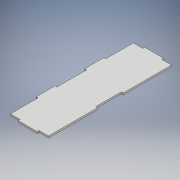
# Autodesk Inventor part: sampingkiri
Saved by Autodesk Inventor 2017 (Build 210142000, 142)
## iProperties
Created: 2017-01-17
Part Number: sampingkiri
Material: Generic
Document SubType Name: Modeling
Designer: Ghesa Bhakti
Density: 1 g/cm^3
Appearance: Default
Author: Ghesa Bhakti
Autodesk Inventor part; units mm, degrees
ref_plane "YZ Plane" through (0, 0, 0) normal (1, 0, 0) x (0, 1, 0)
ref_plane "XZ Plane" through (0, 0, 0) normal (0, 1, 0) x (-1, 0, 0)
ref_plane "XY Plane" through (0, 0, 0) normal (0, 0, 1) x (1, 0, 0)
sketch "Sketch1" plane through (0, 0, 0) normal (0, 0, 1) x (1, 0, 0)
  line L0 (60.0759, 197.5616) -> (45.0759, 197.5616)
  line L1 (45.0759, 197.5616) -> (45.0759, 200.5616)
  line L2 (15.0759, 200.5616) -> (15.0759, 197.5616)
  line L3 (45.0759, 200.5616) -> (15.0759, 200.5616)
  line L4 (15.0759, 197.5616) -> (0.0759, 197.5616)
  line L5 (57.0759, 81.5616) -> (60, 81.5616)
  line L6 (0.0759, 77.6616) -> (-2.9241, 77.6616)
  line L7 (-2.9241, 77.6616) -> (-2.9241, 47.8616)
  line L8 (-2.9241, 47.8616) -> (0.0759, 47.8616)
  line L9 (60, 4.5616) -> (60, 81.5616)
  line L10 (0.0759, 47.8616) -> (0.0759, 4.5616)
  line L11 (0.0759, 4.5616) -> (15.0759, 4.5616)
  line L12 (60.0757, 4.4159) -> (60, 4.5616)
  line L13 (45.0759, 4.4159) -> (60.0757, 4.4159)
  line L14 (45.0759, 4.4159) -> (45.0759, 1.4159)
  line L15 (45.0759, 1.4159) -> (15.0759, 1.5616)
  line L16 (15.0759, 1.5616) -> (15.0759, 4.5616)
  line L17 (0.0759, 197.5616) -> (0.0759, 154.2616)
  line L18 (0.0759, 154.2616) -> (-2.9241, 154.2616)
  line L19 (60.0759, 121.5616) -> (60.0759, 197.5616)
  line L20 (60.0759, 121.5616) -> (57.0759, 121.5616)
  line L21 (-2.9241, 124.2616) -> (0.0759, 124.2616)
  line L22 (-2.9241, 154.2616) -> (-2.9241, 124.2616)
  line L23 (0.0759, 124.2616) -> (0.0759, 77.6616)
  line L24 (57.0759, 121.5616) -> (57.0759, 81.5616)
  point P0 (0, 0)
  dimension "d47" = 193
  dimension "d48" = 60
  dimension "d49" = 3
  dimension "d50" = 30
  dimension "d51" = 15
  dimension "d52" = 3
  dimension "d53" = 3
  dimension "d54" = 15
  dimension "d55" = 3
  dimension "d56" = 3
  dimension "d57" = 3
  dimension "d58" = 3
  dimension "d59" = 15
  dimension "d60" = 40
  dimension "d61" = 3
  dimension "d62" = 77
  dimension "d63" = 3
  dimension "d64" = 76
  dimension "d65" = 199.1457
  dimension "d66" = 43.3
  dimension "d67" = 46.6
  dimension "d68" = 43.3
  dimension "d69" = 30
  dimension "d70" = 29.8
  constraints: 50 end point, 9 parallel, 5 horizontal, 3 perpendicular, 2 vertical, 1 point on line
  measures "d47" distance of L4.end L10.end
  measures "d48" distance of L10.end L12.start
  measures "d49" distance of L0.end L1.end
  measures "d50" distance of L1.end L2.start
  measures "d51" distance of L2.end L4.end
  measures "d52" distance of L18.start L18.end
  measures "d53" distance of L6.start L6.end
  measures "d54" distance of L0.start L0.end
  measures "d55" distance of L8.start L10.start
  measures "d56" distance of L21.start L23.start
  measures "d57" distance of L13.start L14.end
  measures "d58" distance of L16.start L11.end
  measures "d59" distance of L10.end L11.end
  measures "d60" distance of L24.start L5.start
  measures "d61" distance of L20.start L24.start
  measures "d62" distance of L9.start L9.end
  measures "d63" distance of L2.start L2.end
  measures "d64" distance of L20.start L0.start
  measures "d65" distance of L14.end L1.end
  measures "d66" distance of L4.end L18.start
  measures "d67" distance of L23.start L6.start
  measures "d68" distance of L10.start L10.end
  measures "d69" distance of L18.end L21.start
  measures "d70" distance of L6.end L8.start
extrude "Extrusion1" add sketch "Sketch1" along normal blind 3
body "Solid1"
